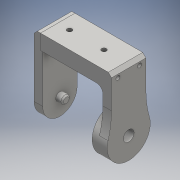
# Autodesk Inventor part: Arm - effector hinge
Saved by Autodesk Inventor 2016 (Build 200138000, 138)
## iProperties
Created: 2016-05-01
Part Number: Arm - effector hinge
Material: Generic
Document SubType Name: Modeling
Designer: Ali
Density: 1 g/cm^3
Appearance: Default
Author: Ali
Autodesk Inventor part; units mm, degrees
ref_plane "YZ Plane" through (0, 0, 0) normal (1, 0, 0) x (0, 1, 0)
ref_plane "XZ Plane" through (0, 0, 0) normal (0, 1, 0) x (-1, 0, 0)
ref_plane "XY Plane" through (0, 0, 0) normal (0, 0, 1) x (1, 0, 0)
sketch "Sketch1" plane through (0, 0, 0) normal (0, 1, 0) x (-1, 0, 0)
  line L0 (0, 9.1892) -> (12.5, 9.1892)
  line L1 (12.5, 9.1892) -> (12.5, -12.6163)
  line L2 (0, -12.6163) -> (0, 13.1892)
  line L3 (16.5, -12.6163) -> (12.5, -12.6163)
  line L4 (0, 13.1892) -> (16.5, 13.1892)
  line L5 (16.5, 13.1892) -> (16.5, -12.6163)
  line L6 (0, 9.1892) -> (-12.5, 9.1892)
  line L7 (-12.5, 9.1892) -> (-12.5, -12.6163)
  line L8 (-16.5, -12.6163) -> (-12.5, -12.6163)
  line L9 (0, 13.1892) -> (-16.5, 13.1892)
  line L10 (-16.5, 13.1892) -> (-16.5, -12.6163)
  point P0 (0, 0)
  dimension "d1" = 4
  dimension "d2" = 4
  constraints: 22 end point, 4 symmetric about line, 3 point on line, 1 parallel, 1 vertical
  measures "d1" distance between parallel lines of L1 L5
  measures "d2" distance between parallel lines of L4 L0
extrude "Extrusion1" add sketch "Sketch1" along normal blind 16
sketch "Sketch2" plane through (16.5, 0, 13.1892) normal (1, 0, 0) x (0, 0, -1)
  line L0 (25.8055, 0) -> (25.8055, 16) projected
  circle A0 centre (25.8055, 8) radius 10
  point P0 (13.1892, 0)
  dimension "d5" = 20
  constraints: 1 centre point, 1 midpoint
  measures "d5" diameter of A0
extrude "Extrusion2" add sketch "Sketch2" against normal blind 7
sketch "Sketch3" plane through (9.5, 8, -12.6163) normal (-1, 0, 0) x (0, 0, 1)
  circle A0 centre (0, 0) radius 10 projected
  circle A1 centre (0, 0) radius 8.825
  point P0 (12.6163, -8)
  dimension "d8" = 17.65
  constraints: 1 centre point, 1 coincident
  measures "d8" diameter of A1
extrude "Extrusion3" cut sketch "Sketch3" against normal blind 2.5 contours A1
sketch "Sketch4" plane through (12, 8, -12.6163) normal (-1, 0, 0) x (0, 0, 1)
  circle A0 centre (0, 0) radius 8.825 projected
  circle A1 centre (-6, 0) radius 1.95
  line L0 (-8.825, 0) -> (8.825, 0) construction
  circle A2 centre (0, -6) radius 1.95
  circle A3 centre (6, 0) radius 1.95
  circle A4 centre (0, 6) radius 1.95
  point P0 (12.6163, -8)
  dimension "d11" = 3.9
  dimension "d12" = 6
  dimension "d15" = 360
  constraints: 4 centre point, 2 end point, 2 point on circle, 1 horizontal, 1 midpoint, 1 point on line, 9 other
  measures "d11" diameter of A1
  measures "d12" distance of A1.centre A0.centre
extrude "Extrusion4" add sketch "Sketch4" along normal blind 3 contours A1 | A2 | A3 | A4
chamfer "Chamfer1" distance 0.6 angle 45 4 edges at (9, 8, -20.5663) (9, 14, -14.5663) (9, 2, -14.5663) (9, 8, -8.5663)
sketch "Sketch5" plane through (-12.5, 0, 9.1892) normal (1, 0, 0) x (0, 0, -1)
  line L0 (0, 0) -> (21.8055, 0) projected
  line L1 (21.8055, 0) -> (21.8055, 16) projected
  line L2 (0, 16) -> (21.8055, 16) projected
  line L3 (0, 0) -> (0, 16) projected
  point P0 (9.1892, 0)
extrude "Extrusion5" cut sketch "Sketch5" against normal through all
sketch "Sketch6" plane through (-16.5, 0, 13.1892) normal (0, 0, 1) x (1, 0, 0)
  line L0 (0, 0) -> (33, 0) projected
  line L1 (33, 0) -> (33, 16) projected
  line L2 (0, 16) -> (33, 16) projected
  line L3 (0, 0) -> (0, 16) projected
  point P0 (16.5, 0)
extrude "Extrusion6" add sketch "Sketch6" along normal blind 3
sketch "Sketch7" plane through (16.5, 8, -12.6163) normal (1, 0, 0) x (0, 0, -1)
  arc A0 (-6, -8) -> (-6, 8) centre (0, 0) ccw projected
  line L0 (-25.8181, 5) -> (-25.8181, -5) construction
  point P0 (-12.6163, -8)
  dimension "d26" = 10
  dimension "d27" = 5
  constraints: 2 end point, 1 vertical
  measures "d26" distance of L0.end L0.start
  measures "d27" vertical distance of A0.centre L0.start
hole "Hole1" at (16.5, 13, 13.2018) at (16.5, 3, 13.2018) direction (-1, 0, 0) diameter 1.9 end through all
sketch "Sketch8" plane through (-16.5, 0, 9.1892) normal (-1, 0, 0) x (0, 0, 1)
  circle A0 centre (4.0126, 13) radius 0.95 projected
  circle A1 centre (4.0126, 3) radius 0.95 projected
  line L0 (0, 16) -> (0, 0) projected
  line L1 (0, 0) -> (7, 0) projected
  line L2 (7, 16) -> (7, 0) projected
  line L3 (0, 16) -> (7, 16) projected
  point P0 (-9.1892, 0)
extrude "Extrusion7" add sketch "Sketch8" along normal blind 3 separate body
sketch "Sketch9" plane through (-16.5, 0, 9.1892) normal (0, 0, -1) x (-1, 0, 0)
  line L0 (0, 16) -> (0, 0) projected
  line L1 (0, 0) -> (3, 0) projected
  line L2 (3, 16) -> (3, 0) projected
  line L3 (0, 16) -> (3, 16) projected
  point P0 (-16.5, 0)
extrude "Extrusion8" add sketch "Sketch9" along normal blind 22 bodies 2
sketch "Sketch10" plane through (-19.5, 0, 9.1892) normal (-1, 0, 0) x (0, 0, 1)
  line L0 (-22, 0) -> (-22, 16) projected
  circle A0 centre (-22, 8) radius 8
  point P0 (-9.1892, 0)
  constraints: 1 midpoint, 1 vertical alignment, 2 other
extrude "Extrusion9" add sketch "Sketch10" against normal blind 4 bodies 2
sketch "Sketch11" plane through (-16.5, 0, 9.1892) normal (1, 0, 0) x (0, 0, -1)
  line L0 (-7, 16) -> (22, 16) projected
  line L1 (-7, 0) -> (22, 0) projected
  arc A0 (22, 0) -> (22, 16) centre (22, 8) ccw projected
  line L2 (0, 0) -> (0, 16) projected
  point P0 (9.1892, 0)
extrude "Extrusion10" add sketch "Sketch11" along normal blind 1 bodies 2
hole "Hole2" at (-19.5, 13, 13.2018) direction (1, 0, 0) diameter 2.1 end through all bodies 2
hole "Hole3" at (-19.5, 3, 13.2018) direction (1, 0, 0) diameter 2.1 end through all bodies 2
sketch "Sketch12" plane through (-15.5, 0, 9.1892) normal (1, 0, 0) x (0, 0, -1)
  arc A0 (22, 0) -> (22, 16) centre (22, 8) ccw projected
  circle A1 centre (22, 8) radius 1.9
  point P0 (9.1892, 0)
  dimension "d61" = 3.8
  constraints: 1 centre point, 1 coincident
  measures "d61" diameter of A1
extrude "Extrusion11" add sketch "Sketch12" along normal blind 3 bodies 2
chamfer "Chamfer2" distance 0.6 angle 45 1 edges at (-12.5, 8, -10.9108)
fillet "Fillet1" radius 3 1 edges at (12.5, 8, 9.1892)
chamfer "Chamfer3" distance 1.5 angle 45 2 edges at (16.5, 8, 16.1892) (-19.5, 8, 16.1892)
fillet "Fillet2" radius 40 2 edges at (14.5, 16, -6.6163) (14.5, 0, -6.6163)
sketch "Sketch13" plane through (-16.5, 0, 16.1892) normal (0, 0, 1) x (1, 0, 0)
  line L0 (1, 24.0112) -> (26, 24.0112) construction
  line L1 (1, 16) -> (1, 0) construction
  line L2 (26, 18) -> (26, -2) construction
  line L3 (13.5, 24.0112) -> (13.5, 8) construction
  line L4 (13.5, 8) -> (5.5, 8) construction
  line L5 (13.5, 8) -> (21.5, 8) construction
  point P0 (16.5, 0)
  point P1 (1, 8)
  dimension "d72" = 16
  constraints: 9 end point, 4 point on line, 3 horizontal, 2 midpoint, 1 collinear, 1 vertical
  measures "d72" distance of L5.end L4.end
hole "Hole4" at (-11, 8, 16.1892) at (5, 8, 16.1892) direction (0, 0, -1) diameter 2.2 end through all bodies 1
sketch "Sketch14" plane through (-16.5, 0, 9.1892) normal (0, 0, -1) x (-1, 0, 0)
  circle A0 centre (-5.5, 8) radius 1.1 projected
  line L0 (-7.6, 6.7876) -> (-7.6, 9.2124)
  line L1 (-7.6, 9.2124) -> (-5.5, 10.4249)
  line L2 (-5.5, 10.4249) -> (-3.4, 9.2124)
  line L3 (-3.4, 9.2124) -> (-3.4, 6.7876)
  line L4 (-3.4, 6.7876) -> (-5.5, 5.5751)
  line L5 (-5.5, 5.5751) -> (-7.6, 6.7876)
  circle A1 centre (-21.5, 8) radius 1.1 projected
  line L6 (-23.6, 6.7876) -> (-23.6, 9.2124)
  line L7 (-23.6, 9.2124) -> (-21.5, 10.4249)
  line L8 (-21.5, 10.4249) -> (-19.4, 9.2124)
  line L9 (-19.4, 9.2124) -> (-19.4, 6.7876)
  line L10 (-19.4, 6.7876) -> (-21.5, 5.5751)
  line L11 (-21.5, 5.5751) -> (-23.6, 6.7876)
  point P0 (-16.5, 0)
  dimension "d80" = 4.2
  dimension "d81" = 4.2
  constraints: 24 end point, 2 coincident, 26 other
  measures "d80" distance between parallel lines of L4 L1
  measures "d81" distance between parallel lines of L8 L11
extrude "Extrusion12" cut sketch "Sketch14" against normal blind 2.5 bodies 1
hole "Hole5" at (16.5, 8, -12.6163) direction (-1, 0, 0) diameter 5 end through all bodies 1
equation "\"d2\" = d1"
equation "\"d27\" = 0.5 * d26"
equation "\"d81\" = d80"
body "Solid1"
body "Solid2"
